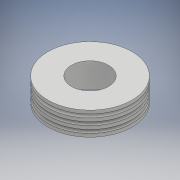
# Autodesk Inventor part: HeatSink-H14p6mm
Saved by Autodesk Inventor 2017 (Build 210142000, 142)
## iProperties
Created: 2022-06-02
Part Number: HeatSink-H14p6mm
Material: Generic
Document SubType Name: Modeling
Designer: Nikita
Density: 1 g/cm^3
Appearance: Default
Author: Nikita
Autodesk Inventor part; units mm, degrees
ref_plane "YZ Plane" through (0, 0, 0) normal (1, 0, 0) x (0, 1, 0)
ref_plane "XZ Plane" through (0, 0, 0) normal (0, 1, 0) x (-1, 0, 0)
ref_plane "XY Plane" through (0, 0, 0) normal (0, 0, 1) x (1, 0, 0)
sketch "Sketch1" plane through (0, 0, 0) normal (0, 1, 0) x (-1, 0, 0)
  line L0 (-11.05, -7.3) -> (11.05, -7.3)
  line L1 (11.05, -7.3) -> (11.05, 7.3)
  line L2 (11.05, 7.3) -> (-11.05, 7.3)
  line L3 (-11.05, 7.3) -> (-11.05, -7.3)
  line L4 (-11.05, -7.3) -> (11.05, 7.3) construction
  line L5 (11.05, -7.3) -> (-11.05, 7.3) construction
  line L6 (0, 3.6568) -> (0, -4.6339)
  line L7 (11.05, 7.3) -> (25.05, 7.3)
  line L8 (25.05, 7.3) -> (25.05, 5.3)
  line L9 (25.05, 5.3) -> (11.05, 5.3)
  line L10 (11.05, 5.3) -> (11.05, 7.3)
  line L11 (11.05, 7.3) -> (13.05, 7.3)
  line L12 (13.05, 7.3) -> (13.05, -7.3)
  line L13 (13.05, -7.3) -> (11.05, -7.3)
  line L14 (11.05, -7.3) -> (11.05, 7.3)
  line L15 (11.05, 1.3) -> (11.05, 3.3)
  line L16 (11.05, 3.3) -> (13.05, 3.3)
  line L17 (25.05, 1.3) -> (11.05, 1.3)
  line L18 (25.05, 3.3) -> (25.05, 1.3)
  line L19 (11.05, 3.3) -> (25.05, 3.3)
  line L20 (11.05, -2.7) -> (11.05, -0.7)
  line L21 (11.05, -0.7) -> (13.05, -0.7)
  line L22 (25.05, -2.7) -> (11.05, -2.7)
  line L23 (25.05, -0.7) -> (25.05, -2.7)
  line L24 (11.05, -0.7) -> (25.05, -0.7)
  line L25 (11.05, -6.7) -> (11.05, -4.7)
  line L26 (11.05, -4.7) -> (13.05, -4.7)
  line L27 (25.05, -6.7) -> (11.05, -6.7)
  line L28 (25.05, -4.7) -> (25.05, -6.7)
  line L29 (11.05, -4.7) -> (25.05, -4.7)
  point P0 (0, 0)
  dimension "d0" = 22.1
  dimension "d1" = 14.6
  dimension "d2" = 14
  dimension "d3" = 2
  dimension "d4" = 2
  dimension "d7" = 4
  constraints: 60 end point, 6 parallel, 3 horizontal, 3 perpendicular, 2 midpoint, 2 vertical, 30 other
  measures "d0" distance of L2.end L1.end
  measures "d1" distance of L1.end L0.end
  measures "d2" distance of L8.end L9.end
  measures "d3" distance of L7.end L8.end
  measures "d4" distance of L12.end L13.end
  measures "d7" distance of L1.end L15.end
revolve "Revolution1" add sketch "Sketch1" angle 360 about axis through (0, 0, 3.6568) along (0, 0, -1) contours L1 L27 L12 L13 | L1 L26 L12 L27 | L7 L12 L9 L1 | L1 L22 L12 L26 | L12 L29 L28 L27 | L9 L12 L16 L1 | L7 L8 L9 L12 | L1 L21 L12 L22 | L16 L12 L17 L1 | L1 L17 L12 L21 | L12 L24 L23 L22 | L19 L18 L17 L12
body "Solid1"
